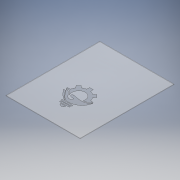
# Autodesk Inventor part: Plaque fond
Saved by Autodesk Inventor 2017 (Build 210142000, 142)
## iProperties
Company: FABLAB Frenchmakers
Part Number: Plaque fond
Project: 1400-PopCorn Machine
Material: Plastique PMMA
Catalog Web Link: http://www.frenchmakers.com/
Document SubType Name: Modeling
Designer: FABLAB Frenchmakers
Density: 1.188 g/cm^3
Appearance: Polycarbonate - Transparent
Stock Number: 1400-04-04
Author: Adrien MARY
Autodesk Inventor part; units mm, degrees
note: some values were not read from the file. Chosen so that the rebuilt part matches the saved one: direction of "Gravure1".
ref_plane "YZ Plane" through (0, 0, 0) normal (1, 0, 0) x (0, 1, 0)
ref_plane "XZ Plane" through (0, 0, 0) normal (0, 1, 0) x (-1, 0, 0)
ref_plane "XY Plane" through (0, 0, 0) normal (0, 0, 1) x (1, 0, 0)
sketch "Esquisse1" plane through (0, 0, 0) normal (0, 0, 1) x (1, 0, 0)
  line L0 (-200.7, -254) -> (200.7, -254)
  line L1 (200.7, -254) -> (200.7, 254)
  line L2 (200.7, 254) -> (-200.7, 254)
  line L3 (-200.7, 254) -> (-200.7, -254)
  line L4 (-200.7, -254) -> (200.7, 254) construction
  line L5 (200.7, -254) -> (-200.7, 254) construction
  point P0 (0, 0)
  dimension "Largueur_plaque_fond" = 401.4
  dimension "Hauteur_plaque_fond" = 508
  constraints: 12 end point, 2 midpoint, 2 parallel, 1 horizontal, 1 perpendicular
  measures "Largueur_plaque_fond" distance of L1.end L2.end
  measures "Hauteur_plaque_fond" distance of L0.end L1.end
extrude "Embase" add sketch "Esquisse1" along normal mid plane 3
sketch "Esquisse3" plane through (0, 0, 1.5) normal (0, 0, 1) x (1, 0, 0)
  line L0 (-22.9723, -70.4472) -> (-24.8203, -71.5651)
  line L1 (-22.693, -70.3539) -> (-22.9723, -70.4472)
  line L2 (-22.3979, -70.2454) -> (-22.693, -70.3539)
  line L3 (-21.0628, -69.997) -> (-22.3979, -70.2454)
  line L4 (-18.7643, -69.9501) -> (-21.0628, -69.997)
  line L5 (-18.0035, -69.9501) -> (-18.7643, -69.9501)
  line L6 (-24.8203, -71.5651) -> (-25.2393, -71.9692)
  line L7 (-17.0562, -69.9501) -> (-18.0035, -69.9501)
  line L8 (-12.9418, -70.2454) -> (-17.0562, -69.9501)
  line L9 (-6.8857, -71.2394) -> (-12.9418, -70.2454)
  line L10 (-4.9607, -71.6118) -> (-6.8857, -71.2394)
  line L11 (-2.0569, -72.1553) -> (-4.9607, -71.6118)
  line L12 (6.7006, -73.7703) -> (-2.0569, -72.1553)
  line L13 (14.744, -75.0588) -> (6.7006, -73.7703)
  line L14 (-26.233, -76.2545) -> (-26.0315, -76.8444)
  line L15 (-23.3143, -81.2854) -> (-22.7084, -81.9068)
  line L16 (-23.6403, -80.9594) -> (-23.3143, -81.2854)
  line L17 (-26.0315, -76.8444) -> (-23.6403, -80.9594)
  line L18 (-32.4442, -86.7047) -> (-36.4504, -82.0928)
  line L19 (-25.2393, -71.9692) -> (-26.2642, -73.6928)
  line L20 (-26.2642, -73.6928) -> (-26.4196, -74.2517)
  line L21 (-26.342, -75.9752) -> (-26.233, -76.2545)
  line L22 (-26.4196, -74.2517) -> (-26.342, -75.9752)
  line L23 (-32.0097, -79.1423) -> (-32.1182, -78.677)
  line L24 (-32.1182, -78.677) -> (-32.6305, -77.7763)
  line L25 (-32.6305, -77.7763) -> (-36.1554, -68.3974)
  line L26 (-37.3975, -72.8851) -> (-35.3789, -75.2454)
  line L27 (-35.3789, -75.2454) -> (-34.5561, -76.2236)
  line L28 (-34.5561, -76.2236) -> (-32.0097, -79.1423)
  line L29 (-62.288, -50.4789) -> (-63.3749, -50.541)
  line L30 (-63.3749, -50.541) -> (-71.356, -50.9603)
  line L31 (-68.2661, -56.9848) -> (-61.6203, -55.9911)
  line L32 (-71.356, -50.9603) -> (-71.4026, -54.6403)
  line L33 (-71.4026, -54.6403) -> (-71.4182, -55.1371)
  line L34 (-69.7722, -57.6837) -> (-68.2661, -56.9848)
  line L35 (-70.8592, -58.3205) -> (-69.7722, -57.6837)
  line L36 (-71.325, -58.3205) -> (-70.8592, -58.3205)
  line L37 (-71.4182, -55.1371) -> (-71.325, -58.3205)
  line L38 (-61.6203, -55.9911) -> (-54.8814, -57.6992)
  line L39 (-62.6762, -61.2238) -> (-63.6855, -61.3328)
  line L40 (-63.6855, -61.3328) -> (-63.9805, -61.3637)
  line L41 (-63.9805, -61.3637) -> (-66.822, -61.9845)
  line L42 (-66.822, -61.9845) -> (-66.822, -62.5749)
  line L43 (-66.822, -62.5749) -> (-65.7506, -63.5223)
  line L44 (-57.3658, -62.4816) -> (-62.6762, -61.2238)
  line L45 (-54.8814, -57.6992) -> (-53.5305, -58.4445)
  line L46 (-53.5305, -58.4445) -> (-52.2106, -59.1743)
  line L47 (-65.0053, -64.3606) -> (-61.1234, -69.1584)
  line L48 (-51.4188, -66.208) -> (-57.3658, -62.4816)
  line L49 (-65.7506, -63.5223) -> (-65.0053, -64.3606)
  line L50 (-35.3168, -49.8424) -> (-28.2361, -36.9238)
  line L51 (-49.4934, -34.1284) -> (-51.2014, -37.4824)
  line L52 (-57.7385, -50.2305) -> (-62.288, -50.4789)
  line L53 (-55.3473, -50.0596) -> (-57.7385, -50.2305)
  line L54 (-54.7106, -47.6841) -> (-55.3473, -50.0596)
  line L55 (-54.6174, -47.3112) -> (-54.7106, -47.6841)
  line L56 (-54.4156, -46.5038) -> (-54.6174, -47.3112)
  line L57 (-51.7293, -38.6627) -> (-54.4156, -46.5038)
  line L58 (-51.4188, -37.995) -> (-51.7293, -38.6627)
  line L59 (-51.2014, -37.4824) -> (-51.4188, -37.995)
  line L60 (-47.6767, -31.0077) -> (-49.4934, -34.1284)
  line L61 (-47.4127, -30.6347) -> (-47.6767, -31.0077)
  line L62 (-46.8226, -29.7344) -> (-47.4127, -30.6347)
  line L63 (-49.0741, -27.2344) -> (-46.8226, -29.7344)
  line L64 (-49.3847, -26.8772) -> (-49.0741, -27.2344)
  line L65 (-31.8231, -14.7502) -> (-33.6554, -13.3839)
  line L66 (-33.6554, -13.3839) -> (-37.1645, -10.3092)
  line L67 (-37.1645, -10.3092) -> (-38.0652, -9.5018)
  line L68 (-38.0652, -9.5018) -> (-44.0588, -4.0983)
  line L69 (-54.0585, -21.6909) -> (-49.3847, -26.8772)
  line L70 (-54.4932, -21.2095) -> (-54.0585, -21.6909)
  line L71 (-57.6608, -17.7004) -> (-54.4932, -21.2095)
  line L72 (-44.0588, -4.0983) -> (-57.6608, -17.7004)
  line L73 (-26.047, -34.8116) -> (-24.6804, -33.4919)
  line L74 (-28.2361, -36.9238) -> (-26.047, -34.8116)
  line L75 (-30.674, -14.0047) -> (-31.8231, -14.7502)
  line L76 (-29.4473, -13.1818) -> (-30.674, -14.0047)
  line L77 (-24.6804, -33.4919) -> (-17.0253, -28.4144)
  line L78 (-13.7955, -6.8625) -> (-22.134, -9.5794)
  line L79 (-12.0411, -6.4896) -> (-13.7955, -6.8625)
  line L80 (-11.5906, -6.3965) -> (-12.0411, -6.4896)
  line L81 (-17.0253, -28.4144) -> (-8.2835, -25.3555)
  line L82 (-8.2835, -25.3555) -> (-6.3734, -25.0449)
  line L83 (-6.3734, -25.0449) -> (-5.7524, -24.9362)
  line L84 (-5.7524, -24.9362) -> (-1.0787, -24.7341)
  line L85 (-1.0787, -24.7341) -> (3.5953, -24.9362)
  line L86 (-22.134, -9.5794) -> (-29.4473, -13.1818)
  line L87 (9.2939, -5.5734) -> (9.0143, -1.117)
  line L88 (-11.2801, -0.5889) -> (-11.5906, -6.3965)
  line L89 (-11.2492, 0.2182) -> (-11.2801, -0.5889)
  line L90 (-10.8768, 7.2212) -> (-11.2492, 0.2182)
  line L91 (-10.7678, 9.2086) -> (-10.8768, 7.2212)
  line L92 (9.0143, -1.117) -> (8.9519, 0.3581)
  line L93 (8.9519, 0.3581) -> (8.9055, 1.1346)
  line L94 (8.455, 9.2086) -> (-10.7678, 9.2086)
  line L95 (8.5795, 7.3609) -> (8.455, 9.2086)
  line L96 (8.9055, 1.1346) -> (8.5795, 7.3609)
  line L97 (20.815, -75.7268) -> (14.744, -75.0588)
  line L98 (25.1939, -75.9598) -> (20.815, -75.7268)
  line L99 (26.6689, -75.9907) -> (25.1939, -75.9598)
  line L100 (29.1535, -76.037) -> (26.6689, -75.9907)
  line L101 (33.5009, -70.0746) -> (33.5009, -70.4939)
  line L102 (33.5475, -50.8982) -> (34.2928, -67.0314)
  line L103 (33.9359, -68.5686) -> (33.5009, -70.0746)
  line L104 (33.5009, -70.4939) -> (35.4264, -70.4315)
  line L105 (40.1777, -75.1518) -> (29.1535, -76.037)
  line L106 (35.4264, -70.4315) -> (38.625, -70.0282)
  line L107 (38.625, -70.0282) -> (39.2616, -69.9346)
  line L108 (39.2616, -69.9346) -> (42.2275, -69.4223)
  line L109 (34.2928, -67.0314) -> (33.9359, -68.5686)
  line L110 (18.1599, -30.2779) -> (27.3364, -38.5228)
  line L111 (27.3364, -38.5228) -> (28.7805, -40.6501)
  line L112 (28.7805, -40.6501) -> (29.1535, -41.1936)
  line L113 (31.172, -44.9048) -> (32.8486, -48.7245)
  line L114 (32.8486, -48.7245) -> (33.0507, -49.3455)
  line L115 (33.0507, -49.3455) -> (33.5475, -50.8982)
  line L116 (29.1535, -41.1936) -> (31.172, -44.9048)
  line L117 (63.4225, -80.0278) -> (64.1056, -78.7854)
  line L118 (61.3882, -83.6766) -> (63.4225, -80.0278)
  line L119 (53.4692, -93.6763) -> (61.3882, -83.6766)
  line L120 (53.5471, -71.084) -> (51.73, -71.8602)
  line L121 (51.73, -71.8602) -> (49.8825, -72.6209)
  line L122 (42.2275, -69.4223) -> (54.8513, -64.3139)
  line L123 (49.8825, -72.6209) -> (40.1777, -75.1518)
  line L124 (62.1804, -65.6027) -> (53.5471, -71.084)
  line L125 (64.1056, -78.7854) -> (69.5867, -64.935)
  line L126 (69.5246, -58.3978) -> (62.1804, -65.6027)
  line L127 (69.5867, -64.935) -> (69.9905, -63.4599)
  line L128 (69.9905, -63.4599) -> (70.1305, -62.8855)
  line L129 (70.1305, -62.8855) -> (71.0309, -58.8792)
  line L130 (70.7204, -56.7828) -> (69.5246, -58.3978)
  line L131 (71.0309, -58.8792) -> (71.5898, -55.8827)
  line L132 (71.5898, -55.8827) -> (70.8288, -56.6279)
  line L133 (70.8288, -56.6279) -> (70.7204, -56.7828)
  line L134 (52.6152, -47.8389) -> (52.2268, -46.2554)
  line L135 (52.6773, -48.1343) -> (52.6152, -47.8389)
  line L136 (53.2051, -50.0596) -> (52.6773, -48.1343)
  line L137 (55.4412, -50.215) -> (53.2051, -50.0596)
  line L138 (59.7579, -50.4634) -> (55.4412, -50.215)
  line L139 (60.7983, -50.5255) -> (59.7579, -50.4634)
  line L140 (61.8232, -50.5719) -> (60.7983, -50.5255)
  line L141 (66.1239, -50.8049) -> (61.8232, -50.5719)
  line L142 (68.3755, -50.9603) -> (66.1239, -50.8049)
  line L143 (66.9628, -52.9634) -> (67.1491, -52.6838)
  line L144 (67.1491, -52.6838) -> (68.3755, -50.9603)
  line L145 (65.1457, -55.3858) -> (66.9628, -52.9634)
  line L146 (54.8513, -64.3139) -> (65.1457, -55.3858)
  line L147 (6.7784, -25.4485) -> (18.1599, -30.2779)
  line L148 (4.2315, -25.0449) -> (6.7784, -25.4485)
  line L149 (3.5953, -24.9362) -> (4.2315, -25.0449)
  line L150 (29.8833, -14.6727) -> (28.7342, -14.1292)
  line L151 (31.7465, -13.0734) -> (29.8833, -14.6727)
  line L152 (35.1626, -10.0608) -> (31.7465, -13.0734)
  line L153 (28.7342, -14.1292) -> (27.383, -13.213)
  line L154 (27.383, -13.213) -> (20.0851, -9.6263)
  line L155 (11.6539, -6.8779) -> (9.8837, -6.4896)
  line L156 (9.8837, -6.4896) -> (9.2939, -5.5734)
  line L157 (20.0851, -9.6263) -> (11.6539, -6.8779)
  line L158 (35.9854, -9.331) -> (35.1626, -10.0608)
  line L159 (41.8703, -4.0208) -> (35.9854, -9.331)
  line L160 (48.6713, -10.8376) -> (41.8703, -4.0208)
  line L161 (45.799, -31.38) -> (44.9601, -30.1224)
  line L162 (44.9601, -30.1224) -> (44.6496, -29.641)
  line L163 (44.6496, -29.641) -> (50.0534, -23.6474)
  line L164 (50.0534, -23.6474) -> (55.4566, -17.6383)
  line L165 (55.4566, -17.6383) -> (48.6713, -10.8376)
  line L166 (52.2268, -46.2554) -> (45.799, -31.38)
  line L167 (-50.0989, -67.3416) -> (-51.4188, -66.208)
  line L168 (-49.4468, -67.9006) -> (-50.0989, -67.3416)
  line L169 (-45.2234, -72.1553) -> (-49.4468, -67.9006)
  line L170 (-52.2106, -59.1743) -> (-45.5027, -64.4227)
  line L171 (-39.2764, -78.8009) -> (-45.2234, -72.1553)
  line L172 (-36.1554, -68.3974) -> (-36.3259, -67.5282)
  line L173 (-36.3259, -67.5282) -> (-36.9006, -64.5314)
  line L174 (-36.9006, -64.5314) -> (-35.3168, -49.8424)
  line L175 (-45.5027, -64.4227) -> (-37.3975, -72.8851)
  line L176 (-23.1122, -95.9278) -> (-23.7957, -95.4001)
  line L177 (-23.7957, -95.4001) -> (-25.7362, -93.7384)
  line L178 (-25.7362, -93.7384) -> (-28.6245, -90.8815)
  line L179 (-28.6245, -90.8815) -> (-32.4442, -86.7047)
  line L180 (-15.5348, -98.5987) -> (-19.2611, -98.024)
  line L181 (-19.2611, -98.024) -> (-22.4445, -96.4401)
  line L182 (-19.0754, -83.8787) -> (-12.9572, -84.7945)
  line L183 (-22.7084, -81.9068) -> (-19.0754, -83.8787)
  line L184 (-22.4445, -96.4401) -> (-23.1122, -95.9278)
  line L185 (-14.2769, -98.5987) -> (-15.5348, -98.5987)
  line L186 (-12.9572, -84.7945) -> (-11.0783, -84.9036)
  line L187 (-11.0783, -84.9036) -> (-10.1155, -84.95)
  line L188 (-5.9081, -97.1081) -> (-12.1965, -98.5987)
  line L189 (-10.1155, -84.95) -> (-6.7309, -85.3223)
  line L190 (-6.7309, -85.3223) -> (-4.5257, -85.9591)
  line L191 (-4.5257, -85.9591) -> (-4.1373, -86.1457)
  line L192 (-1.5601, -94.0646) -> (-5.9081, -97.1081)
  line L193 (-4.1373, -86.1457) -> (-3.4699, -86.4717)
  line L194 (-1.2032, -93.2879) -> (-1.5601, -94.0646)
  line L195 (-3.4699, -86.4717) -> (-1.2495, -89.2665)
  line L196 (-1.2495, -89.2665) -> (-0.939, -92.6517)
  line L197 (-0.939, -92.6517) -> (-1.2032, -93.2879)
  line L198 (-12.1965, -98.5987) -> (-14.2769, -98.5987)
  line L199 (-69.4306, -75.2299) -> (-65.642, -79.6552)
  line L200 (-64.6637, -70.09) -> (-65.2693, -69.7177)
  line L201 (-65.2693, -69.7177) -> (-65.8128, -69.3914)
  line L202 (-65.8128, -69.3914) -> (-71.2008, -68.5686)
  line L203 (-71.2008, -68.5686) -> (-71.6511, -68.7549)
  line L204 (-73.7473, -70.3851) -> (-72.4896, -71.5809)
  line L205 (-73.7473, -69.997) -> (-73.7473, -70.3851)
  line L206 (-73.7473, -69.7017) -> (-73.7473, -69.997)
  line L207 (-71.6511, -68.7549) -> (-73.7473, -69.7017)
  line L208 (-72.4896, -71.5809) -> (-69.4306, -75.2299)
  line L209 (-37.1645, -102.0148) -> (-38.3757, -100.8036)
  line L210 (-35.6428, -103.5365) -> (-37.1645, -102.0148)
  line L211 (-42.3196, -93.3506) -> (-32.0406, -103.8934)
  line L212 (-45.9376, -100.4152) -> (-34.214, -110.0425)
  line L213 (-37.7701, -80.5556) -> (-39.2764, -78.8009)
  line L214 (-36.4504, -82.0928) -> (-37.7701, -80.5556)
  line L215 (-49.9126, -87.1394) -> (-51.6672, -84.8255)
  line L216 (-48.0959, -86.1766) -> (-45.0992, -89.9808)
  line L217 (-45.0992, -89.9808) -> (-44.6023, -90.5867)
  line L218 (-59.3533, -86.8286) -> (-45.9376, -100.4152)
  line L219 (-44.6023, -90.5867) -> (-42.3196, -93.3506)
  line L220 (-43.5774, -95.0895) -> (-49.9126, -87.1394)
  line L221 (-38.3757, -100.8036) -> (-43.5774, -95.0895)
  line L222 (40.6282, -104.4524) -> (53.4692, -93.6763)
  line L223 (25.3799, -112.0144) -> (40.6282, -104.4524)
  line L224 (28.3613, -122.7593) -> (25.3799, -120.3214)
  line L225 (23.2995, -131.1442) -> (22.4143, -130.7249)
  line L226 (23.8118, -131.3771) -> (23.2995, -131.1442)
  line L227 (22.0728, -138.1471) -> (24.8985, -136.9514)
  line L228 (26.2342, -133.6907) -> (23.8118, -131.3771)
  line L229 (26.2342, -134.5447) -> (26.2342, -133.6907)
  line L230 (26.2342, -135.1347) -> (26.2342, -134.5447)
  line L231 (24.8985, -136.9514) -> (26.2342, -135.1347)
  line L232 (-18.3453, -116.0204) -> (-17.3516, -115.8962)
  line L233 (1.0175, -116.3464) -> (7.3374, -116.1291)
  line L234 (-7.3671, -115.8495) -> (-5.939, -116.0358)
  line L235 (-5.939, -116.0358) -> (-5.1313, -116.1446)
  line L236 (-5.1313, -116.1446) -> (1.0175, -116.3464)
  line L237 (-0.3643, -119.7158) -> (-2.7246, -119.7158)
  line L238 (-2.7246, -119.7158) -> (-9.7741, -119.7158)
  line L239 (-9.7741, -119.7158) -> (-17.6312, -119.7316)
  line L240 (-19.1838, -112.4025) -> (-7.3671, -115.8495)
  line L241 (-28.2985, -109.7165) -> (-35.6428, -103.5365)
  line L242 (-22.3049, -110.8653) -> (-20.3015, -111.859)
  line L243 (-20.3015, -111.859) -> (-19.1838, -112.4025)
  line L244 (-17.6312, -119.7316) -> (-23.1432, -119.7782)
  line L245 (-24.541, -115.0421) -> (-19.1684, -116.1137)
  line L246 (-30.8915, -112.1229) -> (-24.541, -115.0421)
  line L247 (-32.1957, -111.3155) -> (-30.8915, -112.1229)
  line L248 (-34.214, -110.0425) -> (-32.1957, -111.3155)
  line L249 (-20.9228, -114.2505) -> (-28.2985, -109.7165)
  line L250 (-32.0406, -103.8934) -> (-22.3049, -110.8653)
  line L251 (-19.3856, -114.9646) -> (-20.9228, -114.2505)
  line L252 (-17.3516, -115.8962) -> (-19.3856, -114.9646)
  line L253 (-19.1684, -116.1137) -> (-18.3453, -116.0204)
  line L254 (25.3799, -120.3214) -> (24.8209, -120.1351)
  line L255 (28.3613, -123.6445) -> (28.3613, -122.7593)
  line L256 (24.8209, -120.1351) -> (23.6564, -119.747)
  line L257 (28.3613, -124.4052) -> (28.3613, -123.6445)
  line L258 (25.6907, -126.7344) -> (28.3613, -124.4052)
  line L259 (25.1784, -126.9517) -> (25.6907, -126.7344)
  line L260 (24.1847, -127.3555) -> (25.1784, -126.9517)
  line L261 (12.57, -115.5081) -> (25.3799, -112.0144)
  line L262 (8.2375, -116.0358) -> (12.57, -115.5081)
  line L263 (7.3374, -116.1291) -> (8.2375, -116.0358)
  line L264 (23.6564, -119.747) -> (-0.3643, -119.7158)
  line L265 (-0.8924, -127.3555) -> (24.1847, -127.3555)
  line L266 (-24.6185, -127.2313) -> (-16.7769, -127.3399)
  line L267 (-24.4165, -130.8491) -> (-24.6028, -130.9113)
  line L268 (-24.6028, -130.9113) -> (-25.2084, -131.0665)
  line L269 (-19.634, -130.7094) -> (-23.2674, -130.7715)
  line L270 (-28.3606, -133.6751) -> (-28.3606, -134.5602)
  line L271 (-25.2084, -131.0665) -> (-28.3606, -133.6751)
  line L272 (-28.3606, -134.5602) -> (-28.3606, -135.1968)
  line L273 (-28.3606, -135.1968) -> (-26.994, -136.9514)
  line L274 (-26.994, -136.9514) -> (-26.6989, -137.1533)
  line L275 (-26.6989, -137.1533) -> (-26.4196, -137.3396)
  line L276 (-26.4196, -137.3396) -> (-25.5032, -137.8676)
  line L277 (-25.5032, -137.8676) -> (-22.8329, -138.2247)
  line L278 (-23.2674, -130.7715) -> (-24.4165, -130.8491)
  line L279 (21.0946, -138.2868) -> (22.0728, -138.1471)
  line L280 (12.3216, -146.5629) -> (10.9705, -142.7898)
  line L281 (10.9705, -142.7898) -> (10.6445, -142.5724)
  line L282 (10.6445, -142.5724) -> (10.0391, -142.1687)
  line L283 (1.6076, -138.411) -> (14.7749, -138.38)
  line L284 (22.4143, -130.7249) -> (-0.6282, -130.6939)
  line L285 (10.0391, -142.1687) -> (-1.0478, -142.1687)
  line L286 (-2.0415, -138.411) -> (1.6076, -138.411)
  line L287 (-1.0478, -142.1687) -> (-3.439, -142.1687)
  line L288 (-0.6282, -130.6939) -> (-3.5941, -130.6783)
  line L289 (-4.8671, -127.3555) -> (-0.8924, -127.3555)
  line L290 (-5.5197, -138.3955) -> (-2.0415, -138.411)
  line L291 (14.7749, -138.38) -> (21.0946, -138.2868)
  line L292 (-7.1965, -152.6652) -> (-6.5755, -152.9913)
  line L293 (-6.5755, -152.9913) -> (-5.6905, -153.4571)
  line L294 (-5.6905, -153.4571) -> (-2.2278, -154.6528)
  line L295 (-2.2278, -154.6528) -> (0.7069, -154.513)
  line L296 (0.7069, -154.513) -> (1.3437, -154.3112)
  line L297 (1.3437, -154.3112) -> (1.7473, -154.1714)
  line L298 (1.7473, -154.1714) -> (3.5953, -153.3795)
  line L299 (12.2283, -147.0133) -> (12.3216, -146.5629)
  line L300 (12.1353, -147.4325) -> (12.2283, -147.0133)
  line L301 (11.2189, -148.9542) -> (12.1353, -147.4325)
  line L302 (8.6571, -150.6467) -> (11.2189, -148.9542)
  line L303 (7.7721, -151.1436) -> (8.6571, -150.6467)
  line L304 (6.7315, -151.7025) -> (7.7721, -151.1436)
  line L305 (3.5953, -153.3795) -> (6.7315, -151.7025)
  line L306 (-16.7769, -127.3399) -> (-4.8671, -127.3555)
  line L307 (-15.9386, -138.3489) -> (-5.5197, -138.3955)
  line L308 (-12.4913, -130.6783) -> (-19.634, -130.7094)
  line L309 (-3.5941, -130.6783) -> (-12.4913, -130.6783)
  line L310 (-3.439, -142.1687) -> (-10.6124, -142.2153)
  line L311 (-10.6124, -142.2153) -> (-12.5534, -142.4171)
  line L312 (-12.5534, -142.4171) -> (-12.6779, -142.4948)
  line L313 (-12.6779, -142.4948) -> (-12.9881, -142.6656)
  line L314 (-12.9881, -142.6656) -> (-14.4168, -145.2276)
  line L315 (-14.4168, -145.2276) -> (-14.4168, -146.0816)
  line L316 (-14.4168, -146.8425) -> (-13.5007, -148.9852)
  line L317 (-14.4168, -146.0816) -> (-14.4168, -146.8425)
  line L318 (-13.5007, -148.9852) -> (-13.2365, -149.2182)
  line L319 (-13.2365, -149.2182) -> (-10.7214, -150.7243)
  line L320 (-10.7214, -150.7243) -> (-7.1965, -152.6652)
  line L321 (-22.8329, -138.2247) -> (-15.9386, -138.3489)
  line L322 (-27.5996, -126.8897) -> (-24.6185, -127.2313)
  line L323 (-28.5469, -126.3617) -> (-27.5996, -126.8897)
  line L324 (-28.8263, -126.1754) -> (-28.5469, -126.3617)
  line L325 (-29.1059, -125.9735) -> (-28.8263, -126.1754)
  line L326 (-23.1432, -119.7782) -> (-25.3017, -119.8091)
  line L327 (-25.3017, -119.8091) -> (-25.4414, -119.8246)
  line L328 (-25.4414, -119.8246) -> (-26.233, -119.9333)
  line L329 (-26.233, -119.9333) -> (-29.2144, -121.2688)
  line L330 (-29.2144, -121.2688) -> (-30.5034, -123.3649)
  line L331 (-30.5034, -123.3649) -> (-30.441, -123.8463)
  line L332 (-30.441, -123.8463) -> (-29.1059, -125.9735)
  line L333 (-52.9249, -79.8567) -> (-48.0959, -86.1766)
  line L334 (-51.6672, -84.8255) -> (-52.9094, -83.1955)
  line L335 (-62.2259, -83.5988) -> (-59.3533, -86.8286)
  line L336 (-63.0954, -82.6206) -> (-62.2259, -83.5988)
  line L337 (-52.9094, -83.1955) -> (-56.6981, -78.3662)
  line L338 (-54.3379, -77.9938) -> (-52.9249, -79.8567)
  line L339 (-55.6733, -76.2082) -> (-54.3379, -77.9938)
  line L340 (-65.642, -79.6552) -> (-63.0954, -82.6206)
  line L341 (-56.6981, -78.3662) -> (-60.2695, -74.096)
  line L342 (-61.1234, -69.1584) -> (-55.6733, -76.2082)
  line L343 (-60.2695, -74.096) -> (-62.9557, -71.4255)
  line L344 (-62.9557, -71.4255) -> (-64.6637, -70.09)
  line L345 (-22.9723, -70.4472) -> (-24.8203, -71.5651)
  line L346 (-22.693, -70.3539) -> (-22.9723, -70.4472)
  line L347 (-22.3979, -70.2454) -> (-22.693, -70.3539)
  line L348 (-21.0628, -69.997) -> (-22.3979, -70.2454)
  line L349 (-18.7643, -69.9501) -> (-21.0628, -69.997)
  line L350 (-18.0035, -69.9501) -> (-18.7643, -69.9501)
  line L351 (-24.8203, -71.5651) -> (-25.2393, -71.9692)
  line L352 (-17.0562, -69.9501) -> (-18.0035, -69.9501)
  line L353 (-12.9418, -70.2454) -> (-17.0562, -69.9501)
  line L354 (-6.8857, -71.2394) -> (-12.9418, -70.2454)
  line L355 (-4.9607, -71.6118) -> (-6.8857, -71.2394)
  line L356 (-2.0569, -72.1553) -> (-4.9607, -71.6118)
  line L357 (6.7006, -73.7703) -> (-2.0569, -72.1553)
  line L358 (14.744, -75.0588) -> (6.7006, -73.7703)
  line L359 (-26.233, -76.2545) -> (-26.0315, -76.8444)
  line L360 (-23.3143, -81.2854) -> (-22.7084, -81.9068)
  line L361 (-23.6403, -80.9594) -> (-23.3143, -81.2854)
  line L362 (-26.0315, -76.8444) -> (-23.6403, -80.9594)
  line L363 (-32.4442, -86.7047) -> (-36.4504, -82.0928)
  line L364 (-25.2393, -71.9692) -> (-26.2642, -73.6928)
  line L365 (-26.2642, -73.6928) -> (-26.4196, -74.2517)
  line L366 (-26.342, -75.9752) -> (-26.233, -76.2545)
  line L367 (-26.4196, -74.2517) -> (-26.342, -75.9752)
  line L368 (-32.0097, -79.1423) -> (-32.1182, -78.677)
  line L369 (-32.1182, -78.677) -> (-32.6305, -77.7763)
  line L370 (-32.6305, -77.7763) -> (-36.1554, -68.3974)
  line L371 (-37.3975, -72.8851) -> (-35.3789, -75.2454)
  line L372 (-35.3789, -75.2454) -> (-34.5561, -76.2236)
  line L373 (-34.5561, -76.2236) -> (-32.0097, -79.1423)
  line L374 (-62.288, -50.4789) -> (-63.3749, -50.541)
  line L375 (-63.3749, -50.541) -> (-71.356, -50.9603)
  line L376 (-68.2661, -56.9848) -> (-61.6203, -55.9911)
  line L377 (-71.356, -50.9603) -> (-71.4026, -54.6403)
  line L378 (-71.4026, -54.6403) -> (-71.4182, -55.1371)
  line L379 (-69.7722, -57.6837) -> (-68.2661, -56.9848)
  line L380 (-70.8592, -58.3205) -> (-69.7722, -57.6837)
  line L381 (-71.325, -58.3205) -> (-70.8592, -58.3205)
  line L382 (-71.4182, -55.1371) -> (-71.325, -58.3205)
  line L383 (-61.6203, -55.9911) -> (-54.8814, -57.6992)
  line L384 (-62.6762, -61.2238) -> (-63.6855, -61.3328)
  line L385 (-63.6855, -61.3328) -> (-63.9805, -61.3637)
  line L386 (-63.9805, -61.3637) -> (-66.822, -61.9845)
  line L387 (-66.822, -61.9845) -> (-66.822, -62.5749)
  line L388 (-66.822, -62.5749) -> (-65.7506, -63.5223)
  line L389 (-57.3658, -62.4816) -> (-62.6762, -61.2238)
  line L390 (-54.8814, -57.6992) -> (-53.5305, -58.4445)
  line L391 (-53.5305, -58.4445) -> (-52.2106, -59.1743)
  line L392 (-65.0053, -64.3606) -> (-61.1234, -69.1584)
  line L393 (-51.4188, -66.208) -> (-57.3658, -62.4816)
  line L394 (-65.7506, -63.5223) -> (-65.0053, -64.3606)
  line L395 (-35.3168, -49.8424) -> (-28.2361, -36.9238)
  line L396 (-49.4934, -34.1284) -> (-51.2014, -37.4824)
  line L397 (-57.7385, -50.2305) -> (-62.288, -50.4789)
  line L398 (-55.3473, -50.0596) -> (-57.7385, -50.2305)
  line L399 (-54.7106, -47.6841) -> (-55.3473, -50.0596)
  line L400 (-54.6174, -47.3112) -> (-54.7106, -47.6841)
  line L401 (-54.4156, -46.5038) -> (-54.6174, -47.3112)
  line L402 (-51.7293, -38.6627) -> (-54.4156, -46.5038)
  line L403 (-51.4188, -37.995) -> (-51.7293, -38.6627)
  line L404 (-51.2014, -37.4824) -> (-51.4188, -37.995)
  line L405 (-47.6767, -31.0077) -> (-49.4934, -34.1284)
  line L406 (-47.4127, -30.6347) -> (-47.6767, -31.0077)
  line L407 (-46.8226, -29.7344) -> (-47.4127, -30.6347)
  line L408 (-49.0741, -27.2344) -> (-46.8226, -29.7344)
  line L409 (-49.3847, -26.8772) -> (-49.0741, -27.2344)
  line L410 (-31.8231, -14.7502) -> (-33.6554, -13.3839)
  line L411 (-33.6554, -13.3839) -> (-37.1645, -10.3092)
  line L412 (-37.1645, -10.3092) -> (-38.0652, -9.5018)
  line L413 (-38.0652, -9.5018) -> (-44.0588, -4.0983)
  line L414 (-54.0585, -21.6909) -> (-49.3847, -26.8772)
  line L415 (-54.4932, -21.2095) -> (-54.0585, -21.6909)
  line L416 (-57.6608, -17.7004) -> (-54.4932, -21.2095)
  line L417 (-44.0588, -4.0983) -> (-57.6608, -17.7004)
  line L418 (-26.047, -34.8116) -> (-24.6804, -33.4919)
  line L419 (-28.2361, -36.9238) -> (-26.047, -34.8116)
  line L420 (-30.674, -14.0047) -> (-31.8231, -14.7502)
  line L421 (-29.4473, -13.1818) -> (-30.674, -14.0047)
  line L422 (-24.6804, -33.4919) -> (-17.0253, -28.4144)
  line L423 (-13.7955, -6.8625) -> (-22.134, -9.5794)
  line L424 (-12.0411, -6.4896) -> (-13.7955, -6.8625)
  line L425 (-11.5906, -6.3965) -> (-12.0411, -6.4896)
  line L426 (-17.0253, -28.4144) -> (-8.2835, -25.3555)
  line L427 (-8.2835, -25.3555) -> (-6.3734, -25.0449)
  line L428 (-6.3734, -25.0449) -> (-5.7524, -24.9362)
  line L429 (-5.7524, -24.9362) -> (-1.0787, -24.7341)
  line L430 (-1.0787, -24.7341) -> (3.5953, -24.9362)
  line L431 (-22.134, -9.5794) -> (-29.4473, -13.1818)
  line L432 (9.2939, -5.5734) -> (9.0143, -1.117)
  line L433 (-11.2801, -0.5889) -> (-11.5906, -6.3965)
  line L434 (-11.2492, 0.2182) -> (-11.2801, -0.5889)
  line L435 (-10.8768, 7.2212) -> (-11.2492, 0.2182)
  line L436 (-10.7678, 9.2086) -> (-10.8768, 7.2212)
  line L437 (9.0143, -1.117) -> (8.9519, 0.3581)
  line L438 (8.9519, 0.3581) -> (8.9055, 1.1346)
  line L439 (8.455, 9.2086) -> (-10.7678, 9.2086)
  line L440 (8.5795, 7.3609) -> (8.455, 9.2086)
  line L441 (8.9055, 1.1346) -> (8.5795, 7.3609)
  line L442 (20.815, -75.7268) -> (14.744, -75.0588)
  line L443 (25.1939, -75.9598) -> (20.815, -75.7268)
  line L444 (26.6689, -75.9907) -> (25.1939, -75.9598)
  line L445 (29.1535, -76.037) -> (26.6689, -75.9907)
  line L446 (33.5009, -70.0746) -> (33.5009, -70.4939)
  line L447 (33.5475, -50.8982) -> (34.2928, -67.0314)
  line L448 (33.9359, -68.5686) -> (33.5009, -70.0746)
  line L449 (33.5009, -70.4939) -> (35.4264, -70.4315)
  line L450 (40.1777, -75.1518) -> (29.1535, -76.037)
  line L451 (35.4264, -70.4315) -> (38.625, -70.0282)
  line L452 (38.625, -70.0282) -> (39.2616, -69.9346)
  line L453 (39.2616, -69.9346) -> (42.2275, -69.4223)
  line L454 (34.2928, -67.0314) -> (33.9359, -68.5686)
  line L455 (18.1599, -30.2779) -> (27.3364, -38.5228)
  line L456 (27.3364, -38.5228) -> (28.7805, -40.6501)
  line L457 (28.7805, -40.6501) -> (29.1535, -41.1936)
  line L458 (31.172, -44.9048) -> (32.8486, -48.7245)
  line L459 (32.8486, -48.7245) -> (33.0507, -49.3455)
  line L460 (33.0507, -49.3455) -> (33.5475, -50.8982)
  line L461 (29.1535, -41.1936) -> (31.172, -44.9048)
  line L462 (63.4225, -80.0278) -> (64.1056, -78.7854)
  line L463 (61.3882, -83.6766) -> (63.4225, -80.0278)
  line L464 (53.4692, -93.6763) -> (61.3882, -83.6766)
  line L465 (53.5471, -71.084) -> (51.73, -71.8602)
  line L466 (51.73, -71.8602) -> (49.8825, -72.6209)
  line L467 (42.2275, -69.4223) -> (54.8513, -64.3139)
  line L468 (49.8825, -72.6209) -> (40.1777, -75.1518)
  line L469 (62.1804, -65.6027) -> (53.5471, -71.084)
  line L470 (64.1056, -78.7854) -> (69.5867, -64.935)
  line L471 (69.5246, -58.3978) -> (62.1804, -65.6027)
  line L472 (69.5867, -64.935) -> (69.9905, -63.4599)
  line L473 (69.9905, -63.4599) -> (70.1305, -62.8855)
  line L474 (70.1305, -62.8855) -> (71.0309, -58.8792)
  line L475 (70.7204, -56.7828) -> (69.5246, -58.3978)
  line L476 (71.0309, -58.8792) -> (71.5898, -55.8827)
  line L477 (71.5898, -55.8827) -> (70.8288, -56.6279)
  line L478 (70.8288, -56.6279) -> (70.7204, -56.7828)
  line L479 (52.6152, -47.8389) -> (52.2268, -46.2554)
  line L480 (52.6773, -48.1343) -> (52.6152, -47.8389)
  line L481 (53.2051, -50.0596) -> (52.6773, -48.1343)
  line L482 (55.4412, -50.215) -> (53.2051, -50.0596)
  line L483 (59.7579, -50.4634) -> (55.4412, -50.215)
  line L484 (60.7983, -50.5255) -> (59.7579, -50.4634)
  line L485 (61.8232, -50.5719) -> (60.7983, -50.5255)
  line L486 (66.1239, -50.8049) -> (61.8232, -50.5719)
  line L487 (68.3755, -50.9603) -> (66.1239, -50.8049)
  line L488 (66.9628, -52.9634) -> (67.1491, -52.6838)
  line L489 (67.1491, -52.6838) -> (68.3755, -50.9603)
  line L490 (65.1457, -55.3858) -> (66.9628, -52.9634)
  line L491 (54.8513, -64.3139) -> (65.1457, -55.3858)
  line L492 (6.7784, -25.4485) -> (18.1599, -30.2779)
  line L493 (4.2315, -25.0449) -> (6.7784, -25.4485)
  line L494 (3.5953, -24.9362) -> (4.2315, -25.0449)
  line L495 (29.8833, -14.6727) -> (28.7342, -14.1292)
  line L496 (31.7465, -13.0734) -> (29.8833, -14.6727)
  line L497 (35.1626, -10.0608) -> (31.7465, -13.0734)
  line L498 (28.7342, -14.1292) -> (27.383, -13.213)
  line L499 (27.383, -13.213) -> (20.0851, -9.6263)
  line L500 (11.6539, -6.8779) -> (9.8837, -6.4896)
  line L501 (9.8837, -6.4896) -> (9.2939, -5.5734)
  line L502 (20.0851, -9.6263) -> (11.6539, -6.8779)
  line L503 (35.9854, -9.331) -> (35.1626, -10.0608)
  line L504 (41.8703, -4.0208) -> (35.9854, -9.331)
  line L505 (48.6713, -10.8376) -> (41.8703, -4.0208)
  line L506 (45.799, -31.38) -> (44.9601, -30.1224)
  line L507 (44.9601, -30.1224) -> (44.6496, -29.641)
  line L508 (44.6496, -29.641) -> (50.0534, -23.6474)
  line L509 (50.0534, -23.6474) -> (55.4566, -17.6383)
  line L510 (55.4566, -17.6383) -> (48.6713, -10.8376)
  line L511 (52.2268, -46.2554) -> (45.799, -31.38)
  line L512 (-50.0989, -67.3416) -> (-51.4188, -66.208)
  line L513 (-49.4468, -67.9006) -> (-50.0989, -67.3416)
  line L514 (-45.2234, -72.1553) -> (-49.4468, -67.9006)
  line L515 (-52.2106, -59.1743) -> (-45.5027, -64.4227)
  line L516 (-39.2764, -78.8009) -> (-45.2234, -72.1553)
  line L517 (-36.1554, -68.3974) -> (-36.3259, -67.5282)
  line L518 (-36.3259, -67.5282) -> (-36.9006, -64.5314)
  line L519 (-36.9006, -64.5314) -> (-35.3168, -49.8424)
  line L520 (-45.5027, -64.4227) -> (-37.3975, -72.8851)
  line L521 (-23.1122, -95.9278) -> (-23.7957, -95.4001)
  line L522 (-23.7957, -95.4001) -> (-25.7362, -93.7384)
  line L523 (-25.7362, -93.7384) -> (-28.6245, -90.8815)
  line L524 (-28.6245, -90.8815) -> (-32.4442, -86.7047)
  line L525 (-15.5348, -98.5987) -> (-19.2611, -98.024)
  line L526 (-19.2611, -98.024) -> (-22.4445, -96.4401)
  line L527 (-19.0754, -83.8787) -> (-12.9572, -84.7945)
  line L528 (-22.7084, -81.9068) -> (-19.0754, -83.8787)
  line L529 (-22.4445, -96.4401) -> (-23.1122, -95.9278)
  line L530 (-14.2769, -98.5987) -> (-15.5348, -98.5987)
  line L531 (-12.9572, -84.7945) -> (-11.0783, -84.9036)
  line L532 (-11.0783, -84.9036) -> (-10.1155, -84.95)
  line L533 (-5.9081, -97.1081) -> (-12.1965, -98.5987)
  line L534 (-10.1155, -84.95) -> (-6.7309, -85.3223)
  line L535 (-6.7309, -85.3223) -> (-4.5257, -85.9591)
  line L536 (-4.5257, -85.9591) -> (-4.1373, -86.1457)
  line L537 (-1.5601, -94.0646) -> (-5.9081, -97.1081)
  line L538 (-4.1373, -86.1457) -> (-3.4699, -86.4717)
  line L539 (-1.2032, -93.2879) -> (-1.5601, -94.0646)
  line L540 (-3.4699, -86.4717) -> (-1.2495, -89.2665)
  line L541 (-1.2495, -89.2665) -> (-0.939, -92.6517)
  line L542 (-0.939, -92.6517) -> (-1.2032, -93.2879)
  line L543 (-12.1965, -98.5987) -> (-14.2769, -98.5987)
  line L544 (-69.4306, -75.2299) -> (-65.642, -79.6552)
  line L545 (-64.6637, -70.09) -> (-65.2693, -69.7177)
  line L546 (-65.2693, -69.7177) -> (-65.8128, -69.3914)
  line L547 (-65.8128, -69.3914) -> (-71.2008, -68.5686)
  line L548 (-71.2008, -68.5686) -> (-71.6511, -68.7549)
  line L549 (-73.7473, -70.3851) -> (-72.4896, -71.5809)
  line L550 (-73.7473, -69.997) -> (-73.7473, -70.3851)
  line L551 (-73.7473, -69.7017) -> (-73.7473, -69.997)
  line L552 (-71.6511, -68.7549) -> (-73.7473, -69.7017)
  line L553 (-72.4896, -71.5809) -> (-69.4306, -75.2299)
  line L554 (-37.1645, -102.0148) -> (-38.3757, -100.8036)
  line L555 (-35.6428, -103.5365) -> (-37.1645, -102.0148)
  line L556 (-42.3196, -93.3506) -> (-32.0406, -103.8934)
  line L557 (-45.9376, -100.4152) -> (-34.214, -110.0425)
  line L558 (-37.7701, -80.5556) -> (-39.2764, -78.8009)
  line L559 (-36.4504, -82.0928) -> (-37.7701, -80.5556)
  line L560 (-49.9126, -87.1394) -> (-51.6672, -84.8255)
  line L561 (-48.0959, -86.1766) -> (-45.0992, -89.9808)
  line L562 (-45.0992, -89.9808) -> (-44.6023, -90.5867)
  line L563 (-59.3533, -86.8286) -> (-45.9376, -100.4152)
  line L564 (-44.6023, -90.5867) -> (-42.3196, -93.3506)
  line L565 (-43.5774, -95.0895) -> (-49.9126, -87.1394)
  line L566 (-38.3757, -100.8036) -> (-43.5774, -95.0895)
  line L567 (40.6282, -104.4524) -> (53.4692, -93.6763)
  line L568 (25.3799, -112.0144) -> (40.6282, -104.4524)
  line L569 (28.3613, -122.7593) -> (25.3799, -120.3214)
  line L570 (23.2995, -131.1442) -> (22.4143, -130.7249)
  line L571 (23.8118, -131.3771) -> (23.2995, -131.1442)
  line L572 (22.0728, -138.1471) -> (24.8985, -136.9514)
  line L573 (26.2342, -133.6907) -> (23.8118, -131.3771)
  line L574 (26.2342, -134.5447) -> (26.2342, -133.6907)
  line L575 (26.2342, -135.1347) -> (26.2342, -134.5447)
  line L576 (24.8985, -136.9514) -> (26.2342, -135.1347)
  line L577 (-18.3453, -116.0204) -> (-17.3516, -115.8962)
  line L578 (1.0175, -116.3464) -> (7.3374, -116.1291)
  line L579 (-7.3671, -115.8495) -> (-5.939, -116.0358)
  line L580 (-5.939, -116.0358) -> (-5.1313, -116.1446)
  line L581 (-5.1313, -116.1446) -> (1.0175, -116.3464)
  line L582 (-0.3643, -119.7158) -> (-2.7246, -119.7158)
  line L583 (-2.7246, -119.7158) -> (-9.7741, -119.7158)
  line L584 (-9.7741, -119.7158) -> (-17.6312, -119.7316)
  line L585 (-19.1838, -112.4025) -> (-7.3671, -115.8495)
  line L586 (-28.2985, -109.7165) -> (-35.6428, -103.5365)
  line L587 (-22.3049, -110.8653) -> (-20.3015, -111.859)
  line L588 (-20.3015, -111.859) -> (-19.1838, -112.4025)
  line L589 (-17.6312, -119.7316) -> (-23.1432, -119.7782)
  line L590 (-24.541, -115.0421) -> (-19.1684, -116.1137)
  line L591 (-30.8915, -112.1229) -> (-24.541, -115.0421)
  line L592 (-32.1957, -111.3155) -> (-30.8915, -112.1229)
  line L593 (-34.214, -110.0425) -> (-32.1957, -111.3155)
  line L594 (-20.9228, -114.2505) -> (-28.2985, -109.7165)
  line L595 (-32.0406, -103.8934) -> (-22.3049, -110.8653)
  line L596 (-19.3856, -114.9646) -> (-20.9228, -114.2505)
  line L597 (-17.3516, -115.8962) -> (-19.3856, -114.9646)
  line L598 (-19.1684, -116.1137) -> (-18.3453, -116.0204)
  line L599 (25.3799, -120.3214) -> (24.8209, -120.1351)
  line L600 (28.3613, -123.6445) -> (28.3613, -122.7593)
  line L601 (24.8209, -120.1351) -> (23.6564, -119.747)
  line L602 (28.3613, -124.4052) -> (28.3613, -123.6445)
  line L603 (25.6907, -126.7344) -> (28.3613, -124.4052)
  line L604 (25.1784, -126.9517) -> (25.6907, -126.7344)
  line L605 (24.1847, -127.3555) -> (25.1784, -126.9517)
  line L606 (12.57, -115.5081) -> (25.3799, -112.0144)
  line L607 (8.2375, -116.0358) -> (12.57, -115.5081)
  line L608 (7.3374, -116.1291) -> (8.2375, -116.0358)
  line L609 (23.6564, -119.747) -> (-0.3643, -119.7158)
  line L610 (-0.8924, -127.3555) -> (24.1847, -127.3555)
  line L611 (-24.6185, -127.2313) -> (-16.7769, -127.3399)
  line L612 (-24.4165, -130.8491) -> (-24.6028, -130.9113)
  line L613 (-24.6028, -130.9113) -> (-25.2084, -131.0665)
  line L614 (-19.634, -130.7094) -> (-23.2674, -130.7715)
  line L615 (-28.3606, -133.6751) -> (-28.3606, -134.5602)
  line L616 (-25.2084, -131.0665) -> (-28.3606, -133.6751)
  line L617 (-28.3606, -134.5602) -> (-28.3606, -135.1968)
  line L618 (-28.3606, -135.1968) -> (-26.994, -136.9514)
  line L619 (-26.994, -136.9514) -> (-26.6989, -137.1533)
  line L620 (-26.6989, -137.1533) -> (-26.4196, -137.3396)
  line L621 (-26.4196, -137.3396) -> (-25.5032, -137.8676)
  line L622 (-25.5032, -137.8676) -> (-22.8329, -138.2247)
  line L623 (-23.2674, -130.7715) -> (-24.4165, -130.8491)
  line L624 (21.0946, -138.2868) -> (22.0728, -138.1471)
  line L625 (12.3216, -146.5629) -> (10.9705, -142.7898)
  line L626 (10.9705, -142.7898) -> (10.6445, -142.5724)
  line L627 (10.6445, -142.5724) -> (10.0391, -142.1687)
  line L628 (1.6076, -138.411) -> (14.7749, -138.38)
  line L629 (22.4143, -130.7249) -> (-0.6282, -130.6939)
  line L630 (10.0391, -142.1687) -> (-1.0478, -142.1687)
  line L631 (-2.0415, -138.411) -> (1.6076, -138.411)
  line L632 (-1.0478, -142.1687) -> (-3.439, -142.1687)
  line L633 (-0.6282, -130.6939) -> (-3.5941, -130.6783)
  line L634 (-4.8671, -127.3555) -> (-0.8924, -127.3555)
  line L635 (-5.5197, -138.3955) -> (-2.0415, -138.411)
  line L636 (14.7749, -138.38) -> (21.0946, -138.2868)
  line L637 (-7.1965, -152.6652) -> (-6.5755, -152.9913)
  line L638 (-6.5755, -152.9913) -> (-5.6905, -153.4571)
  line L639 (-5.6905, -153.4571) -> (-2.2278, -154.6528)
  line L640 (-2.2278, -154.6528) -> (0.7069, -154.513)
  line L641 (0.7069, -154.513) -> (1.3437, -154.3112)
  line L642 (1.3437, -154.3112) -> (1.7473, -154.1714)
  line L643 (1.7473, -154.1714) -> (3.5953, -153.3795)
  line L644 (12.2283, -147.0133) -> (12.3216, -146.5629)
  line L645 (12.1353, -147.4325) -> (12.2283, -147.0133)
  line L646 (11.2189, -148.9542) -> (12.1353, -147.4325)
  line L647 (8.6571, -150.6467) -> (11.2189, -148.9542)
  line L648 (7.7721, -151.1436) -> (8.6571, -150.6467)
  line L649 (6.7315, -151.7025) -> (7.7721, -151.1436)
  line L650 (3.5953, -153.3795) -> (6.7315, -151.7025)
  line L651 (-16.7769, -127.3399) -> (-4.8671, -127.3555)
  line L652 (-15.9386, -138.3489) -> (-5.5197, -138.3955)
  line L653 (-12.4913, -130.6783) -> (-19.634, -130.7094)
  line L654 (-3.5941, -130.6783) -> (-12.4913, -130.6783)
  line L655 (-3.439, -142.1687) -> (-10.6124, -142.2153)
  line L656 (-10.6124, -142.2153) -> (-12.5534, -142.4171)
  line L657 (-12.5534, -142.4171) -> (-12.6779, -142.4948)
  line L658 (-12.6779, -142.4948) -> (-12.9881, -142.6656)
  line L659 (-12.9881, -142.6656) -> (-14.4168, -145.2276)
  line L660 (-14.4168, -145.2276) -> (-14.4168, -146.0816)
  line L661 (-14.4168, -146.8425) -> (-13.5007, -148.9852)
  line L662 (-14.4168, -146.0816) -> (-14.4168, -146.8425)
  line L663 (-13.5007, -148.9852) -> (-13.2365, -149.2182)
  line L664 (-13.2365, -149.2182) -> (-10.7214, -150.7243)
  line L665 (-10.7214, -150.7243) -> (-7.1965, -152.6652)
  line L666 (-22.8329, -138.2247) -> (-15.9386, -138.3489)
  line L667 (-27.5996, -126.8897) -> (-24.6185, -127.2313)
  line L668 (-28.5469, -126.3617) -> (-27.5996, -126.8897)
  line L669 (-28.8263, -126.1754) -> (-28.5469, -126.3617)
  line L670 (-29.1059, -125.9735) -> (-28.8263, -126.1754)
  line L671 (-23.1432, -119.7782) -> (-25.3017, -119.8091)
  line L672 (-25.3017, -119.8091) -> (-25.4414, -119.8246)
  line L673 (-25.4414, -119.8246) -> (-26.233, -119.9333)
  line L674 (-26.233, -119.9333) -> (-29.2144, -121.2688)
  line L675 (-29.2144, -121.2688) -> (-30.5034, -123.3649)
  line L676 (-30.5034, -123.3649) -> (-30.441, -123.8463)
  line L677 (-30.441, -123.8463) -> (-29.1059, -125.9735)
  line L678 (-52.9249, -79.8567) -> (-48.0959, -86.1766)
  line L679 (-51.6672, -84.8255) -> (-52.9094, -83.1955)
  line L680 (-62.2259, -83.5988) -> (-59.3533, -86.8286)
  line L681 (-63.0954, -82.6206) -> (-62.2259, -83.5988)
  line L682 (-52.9094, -83.1955) -> (-56.6981, -78.3662)
  line L683 (-54.3379, -77.9938) -> (-52.9249, -79.8567)
  line L684 (-55.6733, -76.2082) -> (-54.3379, -77.9938)
  line L685 (-65.642, -79.6552) -> (-63.0954, -82.6206)
  line L686 (-56.6981, -78.3662) -> (-60.2695, -74.096)
  line L687 (-61.1234, -69.1584) -> (-55.6733, -76.2082)
  line L688 (-60.2695, -74.096) -> (-62.9557, -71.4255)
  line L689 (-62.9557, -71.4255) -> (-64.6637, -70.09)
  point P0 (-0.8707, -159.327)
  point P1 (-74.3373, -154.5441)
  point P2 (-74.3373, -154.5441)
  constraints: 1380 end point, 28 horizontal, 24 vertical, 1331 other
emboss "Gravure1" sketch "Esquisse3" operation cut depth 0.5 direction (0, 0, -1)
